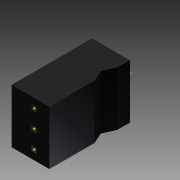
# Autodesk Inventor part: pwm connector
Saved by Autodesk Inventor 2013 (Build 170138000, 138)
## iProperties
Created: 2010-02-11
Part Number: pwm connector
Document SubType Name: Modeling
Designer: Kyle
Density: 1 g/cm^3
Material: Generic
Author: Kyle
Autodesk Inventor part; units mm, degrees
ref_plane "YZ Plane" through (0, 0, 0) normal (1, 0, 0) x (0, 1, 0)
ref_plane "XZ Plane" through (0, 0, 0) normal (0, 1, 0) x (-1, 0, 0)
ref_plane "XY Plane" through (0, 0, 0) normal (0, 0, 1) x (1, 0, 0)
sketch "Sketch1" plane through (0, 0, 0) normal (0, 0, 1) x (1, 0, 0)
  line L0 (2.794, -4.191) -> (2.794, -3.429)
  line L1 (2.794, -3.429) -> (3.556, -3.429)
  line L2 (3.556, -3.429) -> (3.556, -4.191)
  line L3 (3.556, -4.191) -> (2.794, -4.191)
  line L4 (2.794, -6.731) -> (2.794, -5.969)
  line L5 (2.794, -5.969) -> (3.556, -5.969)
  line L6 (3.556, -5.969) -> (3.556, -6.731)
  line L7 (3.556, -6.731) -> (2.794, -6.731)
  line L8 (2.794, -1.651) -> (2.794, -0.889)
  line L9 (2.794, -0.889) -> (3.556, -0.889)
  line L10 (3.556, -0.889) -> (3.556, -1.651)
  line L11 (3.556, -1.651) -> (2.794, -1.651)
  line L12 (5.334, 0) -> (5.334, -7.62)
  line L13 (5.334, 0) -> (0, 0)
  line L14 (0, 0) -> (0, -7.62)
  line L15 (0, -7.62) -> (5.334, -7.62)
  line L16 (5.334, -7.62) -> (6.35, -7.62)
  line L17 (6.35, 0) -> (6.35, -7.62)
  line L18 (6.35, 0) -> (5.334, 0)
  line L19 (-0.611, -8.231) -> (-0.611, 0.611)
  line L20 (-0.611, 0.611) -> (5.334, 0.611)
  line L21 (5.334, 0.611) -> (6.961, 0.611)
  line L22 (6.961, 0.611) -> (6.961, -8.231)
  line L23 (6.961, -8.231) -> (5.334, -8.231)
  line L24 (5.334, -8.231) -> (-0.611, -8.231)
  point P0 (-0.635, 26.67)
  dimension "d2" = 0.611
  constraints: 50 end point, 5 other
  measures "d2" distance between parallel lines of L14 L19
extrude "Extrusion1" add sketch "Sketch1" along normal blind 5.0038 contours L18 L17 L16 L12 | L12 L15 L14 L13
sketch "Sketch2" plane through (0, -7.62, 0) normal (0, -1, 0) x (1, 0, 0)
  point P0 (-0.635, -6.0808)
sketch "Sketch3" plane through (0, -7.62, 0) normal (0, -1, 0) x (1, 0, 0)
  line L0 (6.35, 5.0038) -> (6.35, 0)
  line L1 (5.334, 5.0038) -> (6.35, 5.0038)
  line L2 (4.6228, 3.3857) -> (5.334, 5.0038)
  line L3 (5.334, 1.7675) -> (4.6228, 3.3857)
  line L4 (5.334, 0) -> (5.334, 1.7675)
  line L5 (0, 0) -> (5.334, 0)
  line L6 (5.334, 0) -> (6.35, 0)
  point P0 (-0.635, -6.0808)
  constraints: 14 end point, 1 point on line
extrude "Extrusion2" cut sketch "Sketch3" against normal blind 25.4
ref_plane "Work Plane5" through (0, 0, 8.1788) normal (0, 0, 1) x (1, 0, 0)
ref_plane "Work Plane7" through (0, 0, 11.3538) normal (0, 0, 1) x (1, 0, 0)
ref_plane "Work Plane9" through (0, 0, 8.1788) normal (0, 0, 1) x (1, 0, 0)
ref_plane "Work Plane10" through (0, 0, 11.3538) normal (0, 0, 1) x (1, 0, 0)
ref_plane "Work Plane11" through (0, 0, 8.1788) normal (0, 0, 1) x (1, 0, 0)
ref_plane "Work Plane12" through (0, 0, 11.3538) normal (0, 0, 1) x (1, 0, 0)
sketch "Sketch4" plane through (0, 0, 5.0038) normal (0, 0, 1) x (1, 0, 0)
  line L0 (5.334, -7.62) -> (5.334, 0) projected
  line L1 (0, 0) -> (5.334, 0) projected
  line L2 (0, -7.62) -> (0, 0) projected
  line L3 (5.334, -7.62) -> (0, -7.62) projected
  line L4 (2.794, -3.429) -> (3.556, -3.429) projected
  line L5 (3.556, -3.429) -> (3.556, -4.191) projected
  line L6 (3.556, -4.191) -> (2.794, -4.191) projected
  line L7 (2.794, -4.191) -> (2.794, -3.429) projected
  line L8 (2.794, -5.969) -> (3.556, -5.969) projected
  line L9 (3.556, -5.969) -> (3.556, -6.731) projected
  line L10 (3.556, -6.731) -> (2.794, -6.731) projected
  line L11 (2.794, -6.731) -> (2.794, -5.969) projected
  line L12 (2.794, -0.889) -> (3.556, -0.889) projected
  line L13 (3.556, -0.889) -> (3.556, -1.651) projected
  line L14 (3.556, -1.651) -> (2.794, -1.651) projected
  line L15 (2.794, -1.651) -> (2.794, -0.889) projected
extrude "Extrusion3" add sketch "Sketch4" along normal blind 6.35
ref_plane "Work Plane6" through (0, 0, 8.1788) normal (0, 0, 1) x (1, 0, 0)
ref_plane "Work Plane8" through (0, 0, 11.3538) normal (0, 0, 1) x (1, 0, 0)
body "Solid1"
